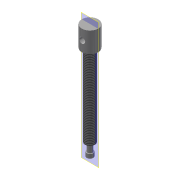
# Autodesk Inventor part: Spindle
Saved by Autodesk Inventor 2022 Beta2 (Build 260130000, 130) ContinuousBuild 0
## iProperties
Created: 2011-02-11
Part Number: Spindle
Material: Generic
Document SubType Name: Modeling
Designer: landrews
Density: 1 g/cm^3
Appearance: Steel
Author: landrews
Autodesk Inventor part; units mm, degrees
ref_plane "YZ Plane" through (0, 0, 0) normal (1, 0, 0) x (0, 1, 0)
ref_plane "XY Plane" through (0, 0, 0) normal (0, 0, 1) x (1, 0, 0)
sketch "Sketch1" plane through (0, 0, 0) normal (1, 0, 0) x (0, 1, 0)
  line L0 (0, 140) -> (10, 140)
  line L1 (10, 140) -> (10, 115)
  line L2 (10, 115) -> (6, 115)
  line L3 (6, 115) -> (6, 15)
  line L4 (3, 5) -> (4, 5)
  line L5 (4, 5) -> (4, 0)
  line L6 (4, 0) -> (0, 0)
  line L7 (0, 168) -> (0, -28) projected
  line L8 (-2, 0) -> (12, 0) projected
  line L9 (3, 5) -> (3, 15)
  line L10 (3, 15) -> (6, 15)
  line L11 (0, 140) -> (0, 0)
  dimension "d4" = 25
  dimension "d8" = 5
  dimension "d9" = 140
  dimension "d12" = 15
  dimension "d15" = 12
  dimension "d16" = 6
  dimension "d17" = 8
  dimension "d18" = 20
  constraints: 20 end point, 5 parallel, 3 perpendicular, 2 point on line, 1 collinear
  measures "d4" distance between parallel lines of L0 L2
  measures "d8" distance between parallel lines of L6 L4
  measures "d9" distance between parallel lines of L8 L0
  measures "d12" distance from line of L8 L3.end
  measures "d15" diameter of L3 L11
  measures "d16" diameter of L9 L7
  measures "d17" diameter of L5 L7
  measures "d18" diameter of L1 L11
revolve "Revolution1" add sketch "Sketch1" angle 360 about axis through (0, 0, 140) along (0, 0, -1)
ref_plane "Work Plane1" through (0, -10, 127.5) normal (0, 1, 0) x (-1, 0, 0)
sketch "Sketch2" plane through (0, -10, 127.5) normal (0, 1, 0) x (-1, 0, 0)
  line L0 (0, -155.5) -> (0, 40.5) projected
  line L1 (-10, 12.5) -> (10, 12.5) projected
  point P0 (0, -127.5)
  point P1 (0, 0)
  dimension "d20" = 12.5
  constraints: 1 point on line
  measures "d20" distance from line of L1 point (0, 0)
hole "Hole1" at (0, -10, 127.5) direction (0, 1, 0) diameter 7 end through all
thread "Thread1" size "M12x1.75" class "6g" standard "ANSI Metric M Profile" full length
body "Solid1"
